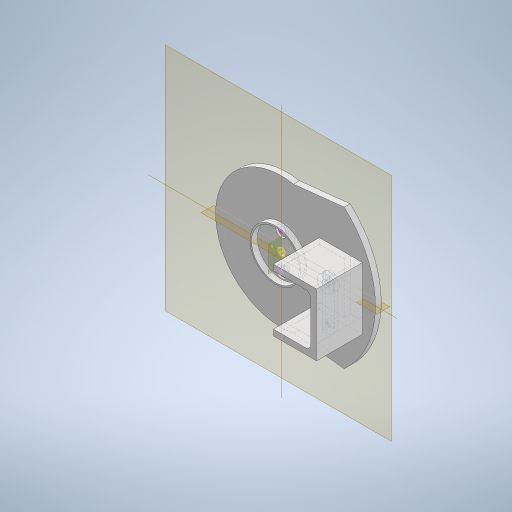
# Autodesk Inventor part: TopGearPlate
Saved by Autodesk Inventor 2023.2 (Build 272271030, 271C)
## iProperties
Created: 2023-06-03
Part Number: TopGearPlate
Material: Generic
Document SubType Name: Modeling
Designer: atrus
Density: 1 g/cm^3
Appearance: Default
Author: atrus
Autodesk Inventor part; units mm, degrees
ref_plane "YZ Plane" through (0, 0, 0) normal (1, 0, 0) x (0, 1, 0)
ref_plane "XZ Plane" through (0, 0, 0) normal (0, 1, 0) x (-1, 0, 0)
ref_plane "Work Plane1" through (0, 0, 0) normal (0, 0, 1) x (1, 0, 0)
sketch "Sketch1" plane through (0, 0, 0) normal (0, 0, 1) x (1, 0, 0)
  circle A0 centre (7.5, 0) radius 3.175 projected
  circle A1 centre (7.5, 15) radius 2.5 construction
  circle A2 centre (7.5, -15) radius 2.5 construction
  arc A3 (69.3283, 4.3421) -> (-40.362, 3.8938) centre (14.5, 0) ccw construction
  arc A4 (17.9696, 54.8905) -> (17.9696, -54.8905) centre (7.5, 0) ccw
  arc A5 (60.9943, -59.4841) -> (60.9943, 59.4841) centre (7.5, 0) ccw projected
  line L0 (60.9943, 59.4841) -> (17.9696, 54.8905)
  line L1 (60.9943, -59.4841) -> (17.9696, -54.8905)
  point P0 (0, 0)
  dimension "d0" = 55.88
  constraints: 4 end point, 3 point on circle, 1 centre point, 1 coincident, 1 equal length
  measures "d0" radius of A4
extrude "Primary Shaft Bore" add sketch "Sketch1" along normal blind 5
sketch "Sketch2" plane through (0, 0, 5) normal (0, 0, 1) x (1, 0, 0)
  circle A0 centre (7.5, 0) radius 3.175 construction
  circle A1 centre (7.5, 0) radius 3.175 projected
  circle A2 centre (7.5, 0) radius 20.32
  circle A3 centre (7.5, 0) radius 21.59
  point P0 (0, 0)
  dimension "d3" = 40.64
  dimension "d4" = 43.18
  constraints: 2 centre point, 2 coincident
  measures "d3" diameter of A2
  measures "d4" diameter of A3
extrude "Large Gear Seat" add sketch "Sketch2" along normal blind 5 contours A3
sketch "Sketch4" plane through (0, 0, 0) normal (0, 0, -1) x (-1, 0, 0)
  circle A0 centre (-7.5, 15) radius 2.5 construction
  circle A1 centre (-7.5, -15) radius 2.5 construction
  point P0 (0, 0)
ref_plane "Work Plane2" through (-496.14, 0, 5) normal (0, 1, 0) x (0, 0, -1)
sketch "Sketch5" plane through (0, 0, 5) normal (0, 0, 1) x (1, 0, 0)
  circle A0 centre (7.5, 0) radius 3.175 projected
  circle A1 centre (7.5, 15) radius 1.5 projected
  circle A2 centre (7.5, -15) radius 1.5 projected
  point P0 (0, 0)
ref_plane "Work Plane5" through (7.5, 0, 5) normal (-1, 0, 0) x (0, -1, 0)
sketch "Sketch7" plane through (0, 0, 5) normal (0, 0, 1) x (1, 0, 0)
  arc A0 (51.7179, -2) -> (48.3952, -2) centre (50.0565, 0) ccw construction
  circle A1 centre (50.0565, 0) radius 6.985
  point P0 (0, 0)
  dimension "d17" = 13.97
  constraints: 1 centre point, 1 coincident
  measures "d17" diameter of A1
extrude "Second Gear Seat" add sketch "Sketch7" along normal up to surface (5 mm away)
sketch "Sketch8" plane through (0, 0, 5) normal (0, 0, 1) x (1, 0, 0)
  point P0 (0, 0)
  point P1 (7.5, 15)
  point P2 (7.5, -15)
hole "Hole1" at (7.5, 15, 5) at (7.5, -15, 5) direction (0, 0, -1) diameter 4.4958 end through all counterbore diameter 9.398 counterbore depth 1.5875 clearance for "Flat Head Machine Screw" size "M4" standard "Ansi Metric M Profile"
sketch "Sketch9" plane through (50.0565, 0, 10) normal (0, 0, 1) x (1, 0, 0)
  arc A0 (1.6613, -2) -> (-1.6613, -2) centre (0, 0) ccw construction
  circle A1 centre (0, 0) radius 2.75
  point P0 (-50.0565, 0)
  dimension "d27" = 5.5
  constraints: 1 centre point, 1 coincident
  measures "d27" diameter of A1
extrude "Extrusion7" cut sketch "Sketch9" against normal blind 6
sketch "Sketch10" plane through (0, 0, 5) normal (0, 0, 1) x (1, 0, 0)
  line L0 (114.676, 0) -> (-75.556, 0) construction
  line L1 (71.4406, -11.5878) -> (71.4406, 11.4122) construction
  line L2 (61.7906, 21.0622) -> (38.7906, 21.0622) construction
  line L3 (38.7906, -21.2378) -> (61.7906, -21.2378) construction
  line L4 (67.587, -21.0914) -> (71.2941, -17.3843) construction
  line L5 (71.2941, 17.2086) -> (67.587, 20.9157) construction
  line L6 (39.7906, -21.4378) -> (68.6548, -21.4378)
  line L7 (68.6548, -21.4378) -> (71.5406, -18.552)
  line L8 (71.5406, -18.552) -> (71.5406, 0)
  line L9 (39.7906, -21.4378) -> (39.7906, -26.4378)
  line L10 (39.7906, -26.4378) -> (76.5406, -26.4378)
  line L11 (76.5406, -26.4378) -> (76.5406, 0)
  line L12 (39.7906, 21.4378) -> (68.6548, 21.4378)
  line L13 (68.6548, 21.4378) -> (71.5406, 18.552)
  line L14 (71.5406, 18.552) -> (71.5406, 0)
  line L15 (39.7906, 21.4378) -> (39.7906, 26.4378)
  line L16 (39.7906, 26.4378) -> (76.5406, 26.4378)
  line L17 (76.5406, 26.4378) -> (76.5406, 0)
  point P0 (0, 0)
  dimension "d30" = 0.2
  dimension "d31" = 0.1
  dimension "d32" = 5
  dimension "d33" = 5
  dimension "d34" = 1
  dimension "d35" = 1
  constraints: 24 end point, 5 symmetric about line, 3 perpendicular, 2 parallel, 2 point on line, 1 horizontal, 1 vertical
  measures "d30" distance between parallel lines of L3 L6
  measures "d31" distance between parallel lines of L8 L1
  measures "d32" distance between parallel lines of L11 L8
  measures "d33" distance between parallel lines of L6 L10
  measures "d34" distance between parallel lines of L4 L7
  measures "d35" distance from line of L9 L3.start
ref_plane "Work Plane6" through (29.6406, -20.7378, 44) normal (0, 0, 1) x (1, 0, 0)
extrude "Extrusion8" add sketch "Sketch10" along normal up to surface (39 mm away)
sketch "Sketch11" plane through (71.5406, -18.552, 5) normal (-1, 0, 0) x (0, 0, 1)
  line L0 (0, -2.8858) -> (39, -2.8858) projected
  line L1 (18.9, -2.8858) -> (16.36, -2.8858)
  line L2 (16.36, -2.8858) -> (16.36, 40.2564)
  line L3 (16.36, 40.2564) -> (18.9, 40.2564)
  line L4 (18.9, 40.2564) -> (18.9, -2.8858)
  line L5 (19, 35.4071) -> (19, 1.5213) construction
  point P0 (-5, 18.552)
  dimension "d38" = 2.54
  dimension "d39" = 0.1
  constraints: 8 end point, 2 parallel, 1 horizontal, 1 perpendicular, 1 point on line
  measures "d38" distance between parallel lines of L2 L4
  measures "d39" distance between parallel lines of L4 L5
extrude "Extrusion9" add sketch "Sketch11" along normal blind 10.16
sketch "Sketch12" plane through (0, 0, 0) normal (0, 0, -1) x (-1, 0, 0)
  line L0 (-61.3806, 21.4378) -> (-61.3806, -21.4378) projected
  line L1 (-39.7906, -21.4378) -> (-68.6548, -21.4378) projected
  line L2 (-68.6548, -21.4378) -> (-71.5406, -18.552) projected
  line L3 (-71.5406, -18.552) -> (-71.5406, 18.552) projected
  line L4 (-71.5406, 18.552) -> (-68.6548, 21.4378) projected
  line L5 (-68.6548, 21.4378) -> (-39.7906, 21.4378) projected
  point P0 (0, 0)
extrude "Extrusion10" cut sketch "Sketch12" against normal blind 10.16
sketch "Sketch13" plane through (71.5406, -18.552, 21.36) normal (0, 0, -1) x (-1, 0, 0)
  circle A0 centre (5.75, 2.9642) radius 2.4 construction
  circle A1 centre (5.75, 33.9642) radius 2.4 construction
  point P0 (71.5406, 18.552)
hole "Hole2" at (65.7906, -15.5878, 21.36) at (65.7906, 15.4122, 21.36) direction (0, 0, 1) diameter 3.4036 end through all countersink diameter 6.2992 countersink angle 90 clearance for "Flat Head Machine Screw" size "M3" standard "Ansi Metric M Profile"
body "Solid1"
